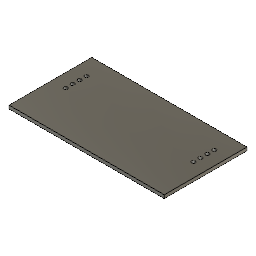
Extension_long_side v9 (Autodesk Fusion 360 design; units mm, degrees)
Autodesk Fusion 360 part; units mm, degrees
sketch "long_side" plane through (0, 0, 0) normal (0, 0, 1) x (1, 0, 0)
  line L0 (0, 152.4) -> (285.75, 152.4)
  line L1 (285.75, 152.4) -> (285.75, 0)
  line L2 (285.75, 0) -> (0, 0)
  line L3 (0, 0) -> (0, 152.4)
  circle A0 centre (25.4, 117.4) radius 3.302
  circle A1 centre (25.4, 92) radius 3.302
  circle A2 centre (25.4, 79.3) radius 3.302
  circle A3 centre (25.4, 104.7) radius 3.302
  circle A4 centre (260.35, 117.4) radius 3.302
  circle A5 centre (260.35, 92) radius 3.302
  circle A6 centre (260.35, 104.7) radius 3.302
  circle A7 centre (260.35, 79.3) radius 3.302
  dimension "d1" = 285.75
  dimension "d2" = 152.4
  dimension "d3" = 6.604
  dimension "d55" = 6.604
  dimension "d57" = 6.604
  dimension "d63" = 6.604
  dimension "d75" = 35
  dimension "d76" = 25.4
  dimension "d77" = 12.7
  dimension "d78" = 25.4
  dimension "d79" = 25.4
  dimension "d80" = 25.4
  dimension "d81" = 12.7
  dimension "d82" = 12.7
  dimension "d89" = 6.604
  dimension "d90" = 6.604
  dimension "d91" = 6.604
  dimension "d92" = 6.604
  dimension "d93" = 12.7
  dimension "d94" = 12.7
  dimension "d95" = 12.7
  dimension "d96" = 25.4
  dimension "d97" = 25.4
  dimension "d98" = 25.4
  dimension "d99" = 25.4
  dimension "d100" = 35
  constraint horizontal L0
  constraint vertical L1
  constraint horizontal L2
  constraint coincident L2.end L3.start
  constraint vertical L3
  measures "d1" distance of L0.start L0.end
  measures "d2" distance of L0.start L2.end
  measures "d3" diameter of A0
  measures "d55" diameter of A1
  measures "d57" diameter of A2
  measures "d63" diameter of A3
  measures "d75" distance of L0 A0.centre
  measures "d76" distance of L3 A0.centre
  measures "d77" distance of A0.centre A3.centre
  measures "d78" distance of L3 A3.centre
  measures "d79" distance of L3 A1.centre
  measures "d80" distance of L3 A2.centre
  measures "d81" distance of A1.centre A3.centre
  measures "d82" distance of A1.centre A2.centre
  measures "d89" diameter of A4
  measures "d90" diameter of A5
  measures "d91" diameter of A7
  measures "d92" diameter of A6
  measures "d93" distance of A4.centre A6.centre
  measures "d94" distance of A6.centre A5.centre
  measures "d95" distance of A7.centre A5.centre
  measures "d96" distance of L1 A4.centre
  measures "d97" distance of L1 A6.centre
  measures "d98" distance of L1 A5.centre
  measures "d99" distance of L1 A7.centre
  measures "d100" distance of L0 A4.centre
extrude "Extrude1" add sketch "long_side" along normal blind 6.35
sketch "Sketch2" plane through (0, 0, 0) normal (0, 0, 1) x (1, 0, 0)
  line L0 (25, 117) -> (25, 104.3) construction
  dimension "d35" = 12.7
  constraint vertical L0
  measures "d35" distance of L0.start L0.end
